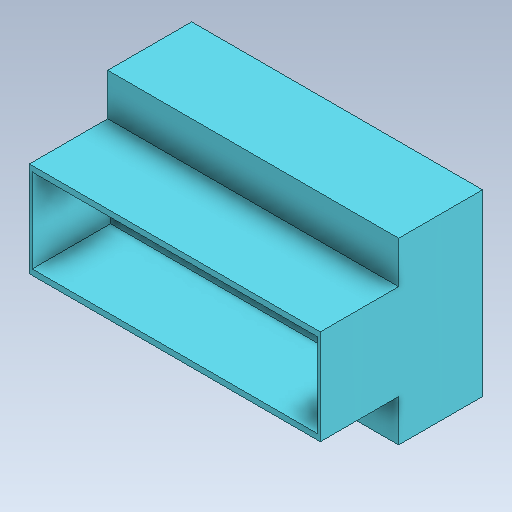
# Autodesk Inventor part: Magazynek na baterie
Saved by Autodesk Inventor 2020 (Build 240168000, 168)
## iProperties
Created: 2021-10-14
Part Number: Magazynek na baterie
Material: Ogólny
Document SubType Name: Modeling
Designer: Komputer
Density: 1 g/cm^3
Appearance: Niebieska z odcieniem szarości
Mass: 5.206 g
Surface Area: 133.24 cm^2
Volume: 5.206 cm^3
Author: Komputer
Autodesk Inventor part; units mm, degrees
ref_plane "YZ Plane" through (0, 0, 0) normal (1, 0, 0) x (0, 1, 0)
ref_plane "XZ Plane" through (0, 0, 0) normal (0, 1, 0) x (-1, 0, 0)
ref_plane "XY Plane" through (0, 0, 0) normal (0, 0, 1) x (1, 0, 0)
sketch "Szkic1" plane through (0, 0, 0) normal (0, 0, 1) x (1, 0, 0)
  line L0 (25.5, -15.5) -> (-25.5, -15.5)
  line L1 (-25.5, -15.5) -> (-25.5, 15.5)
  line L2 (-25.5, 15.5) -> (25.5, 15.5)
  line L3 (25.5, 15.5) -> (25.5, -15.5)
  line L4 (25.5, -15.5) -> (-25.5, 15.5) construction
  line L5 (-25.5, -15.5) -> (25.5, 15.5) construction
  line L6 (26, -16) -> (-26, -16)
  line L7 (-26, -16) -> (-26, 16)
  line L8 (-26, 16) -> (26, 16)
  line L9 (26, 16) -> (26, -16)
  line L10 (26, -16) -> (-26, 16) construction
  line L11 (-26, -16) -> (26, 16) construction
  point P0 (0, 0)
  dimension "d0" = 51
  dimension "d1" = 31
  dimension "d2" = 52
  dimension "d3" = 32
  constraints: 24 end point, 4 midpoint, 4 parallel, 2 horizontal, 2 perpendicular
  measures "d0" distance of L1.end L2.end
  measures "d1" distance of L0.end L1.end
  measures "d2" distance of L7.end L8.end
  measures "d3" distance of L6.end L7.end
extrude "Wyciągnięcie proste1" add sketch "Szkic1" along normal blind 15
sketch "Szkic2" plane through (0, 0, 15) normal (0, 0, 1) x (1, 0, 0)
  line L0 (-25.5, -15.5) -> (-25.5, 15.5) projected
  line L1 (25.5, -15.5) -> (-25.5, -15.5)
  line L2 (-25.5, -15.5) -> (-25.5, 15.5)
  line L3 (-25.5, 15.5) -> (25.5, 15.5)
  line L4 (25.5, 15.5) -> (25.5, -15.5)
  line L5 (25.5, -15.5) -> (-25.5, 15.5) construction
  line L6 (-25.5, -15.5) -> (25.5, 15.5) construction
  point P0 (0, 0)
  constraints: 12 end point, 2 midpoint, 2 parallel, 1 horizontal, 1 perpendicular
extrude "Wyciągnięcie proste2" add sketch "Szkic2" against normal blind 1
sketch "Szkic4" plane through (0, 0, 14) normal (0, 0, -1) x (-1, 0, 0)
  line L0 (-25.5, -15.5) -> (-25.5, 15.5) projected
  line L1 (-25.5, 0) -> (-25.5, 0.5)
  line L2 (-25.5, 0.5) -> (25.5, 0.5)
  line L3 (25.5, 15.5) -> (25.5, -15.5) projected
  line L4 (25.5, -0.5) -> (-25.5, -0.5)
  point P0 (0, 0)
  dimension "d14" = 0.5
  constraints: 6 end point, 4 point on line, 2 perpendicular, 1 midpoint
  measures "d14" distance of L1.start L1.end
extrude "Wyciągnięcie proste4" add sketch "Szkic4" along normal blind 14
sketch "Szkic5" plane through (0, 0, 15) normal (0, 0, 1) x (1, 0, 0)
  line L0 (0, 0) -> (0, 7.5)
  line L1 (0, 7.5) -> (0, 8.5)
  line L2 (0, 8.5) -> (26, 8.5)
  line L3 (26, -16) -> (26, 16) projected
  line L4 (0, 8.5) -> (-26, 8.5)
  line L5 (-26, 16) -> (-26, -16) projected
  line L6 (25.5, -0.5) -> (-25.5, -0.5) projected
  line L7 (0, 0) -> (0, -7.5)
  line L8 (0, -7.5) -> (26, -7.5)
  line L9 (0, -7.5) -> (-26, -7.5)
  line L10 (0, 7.5) -> (26, 7.5)
  line L11 (26, 8.5) -> (26, 7.5)
  line L12 (0, 7.5) -> (-26, 7.5)
  line L13 (-26, 8.5) -> (-26, 7.5)
  line L14 (-26, -7.5) -> (-26, -8.5)
  line L15 (-26, -8.5) -> (26, -8.5)
  line L16 (26, -7.5) -> (26, -8.5)
  line L17 (26, -7.5) -> (26, 7.5)
  line L18 (-26, 7.5) -> (-26, -7.5)
  dimension "d17" = 7.5
  dimension "d18" = 1
  dimension "d20" = 7.5
  dimension "d21" = 1
  constraints: 32 end point, 10 point on line, 5 collinear, 4 perpendicular, 2 horizontal, 2 vertical
  measures "d17" distance of L0.start L0.end
  measures "d18" distance of L0.end L1.end
  measures "d20" distance of L0.start L7.end
  measures "d21" distance of L9.end L14.end
extrude "Wyciągnięcie proste5" add sketch "Szkic5" along normal blind 14 contours L12 L5 L4 L1 | L1 L2 L3 L10 | L8 L3 L15 L5 L9
sketch "Szkic7" plane through (0, 0, 15) normal (0, 0, 1) x (1, 0, 0)
  line L0 (26, 7.5) -> (-26, 7.5) projected
  line L1 (-26, 7.5) -> (-25.5, 7.5)
  line L2 (-25.5, 7.5) -> (-25.5, -7.5)
  line L3 (-25.5, -15.5) -> (-25.5, -0.5) projected
  line L4 (26, -7.5) -> (-26, -7.5) projected
  line L5 (-25.5, -7.5) -> (-26, -7.5)
  line L6 (-26, 8.5) -> (-26, 7.5) projected
  line L7 (-26, -7.5) -> (-26, 7.5)
  line L8 (26, 7.5) -> (25.5, 7.5)
  line L9 (25.5, 15.5) -> (25.5, 0.5) projected
  line L10 (25.5, 7.5) -> (25.5, -7.5)
  line L11 (25.5, -0.5) -> (25.5, -15.5) projected
  line L12 (25.5, -7.5) -> (26, -7.5)
  line L13 (26, -7.5) -> (26, 7.5)
  line L14 (26, -16) -> (26, 16) projected
  point P0 (0, 0)
  point P1 (25.5, 0.5)
  dimension "d30" = 0.5
  dimension "d31" = 15
  constraints: 16 end point, 6 point on line, 3 collinear
  measures "d30" distance of L0.end L1.end
  measures "d31" distance of L1.end L2.end
extrude "Wyciągnięcie proste7" add sketch "Szkic7" along normal blind 14 contours L13 L4 L10 L9 L0 | L2 L4 L7 L0
